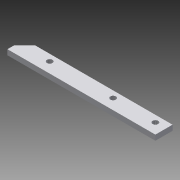
# Autodesk Inventor part: gusset guard
Saved by Autodesk Inventor 2015 (Build 190159000, 159)
## iProperties
Created: 2015-03-29
Part Number: gusset guard
Material: Aluminum 6061
Document SubType Name: Modeling
Designer: Jarod
Density: 2.7 g/cm^3
Appearance: Aluminum - Flat
Author: Jarod
Autodesk Inventor part; units mm, degrees
ref_plane "YZ Plane" through (0, 0, 0) normal (1, 0, 0) x (0, 1, 0)
ref_plane "XZ Plane" through (0, 0, 0) normal (0, 1, 0) x (-1, 0, 0)
ref_plane "XY Plane" through (0, 0, 0) normal (0, 0, 1) x (1, 0, 0)
sketch "Sketch1" plane through (0, 0, 0) normal (0, 1, 0) x (-1, 0, 0)
  line L0 (0, 0) -> (165.1, 0)
  line L1 (177.8, 12.7) -> (177.8, 20.6375)
  line L2 (177.8, 20.6375) -> (0, 20.6375)
  line L3 (0, 20.6375) -> (0, 0)
  line L4 (165.1, 0) -> (177.8, 12.7)
  circle A0 centre (139.7, 7.9375) radius 3.3734
  circle A1 centre (63.5, 7.9375) radius 3.3734
  circle A2 centre (12.7, 7.9375) radius 3.3734
  point P0 (177.8, 0)
  dimension "d0" = 177.8
  dimension "d1" = 20.6375
  dimension "d2" = 12.7
  dimension "d3" = 12.7
  dimension "d4" = 12.7
  dimension "d5" = 12.7
  dimension "d6" = 12.7
  dimension "d7" = 12.7
  dimension "d8" = 63.5
  dimension "d9" = 139.7
  dimension "d10" = 6.7469
  dimension "d11" = 6.7469
  dimension "d12" = 6.7469
  constraints: 10 end point, 3 centre point, 3 coincident, 2 parallel, 2 point on line, 1 horizontal, 1 perpendicular
  measures "d0" distance of L2.end L1.end
  measures "d1" distance of L1.end point (177.8, 0)
  measures "d2" distance of L0.end point (177.8, 0)
  measures "d3" distance of L1.start point (177.8, 0)
  measures "d4" distance from line of L2 point (139.7, 7.938)
  measures "d5" distance from line of L2 point (63.5, 7.938)
  measures "d6" distance from line of L2 point (12.7, 7.938)
  measures "d7" distance from line of L3 point (12.7, 7.938)
  measures "d8" distance from line of L3 point (63.5, 7.938)
  measures "d9" distance from line of L3 point (139.7, 7.938)
  measures "d10" diameter of A0
  measures "d11" diameter of A1
  measures "d12" diameter of A2
extrude "Extrusion1" add sketch "Sketch1" along normal blind 6.35
equation "\"d3\" = d2"
body "Solid1"
